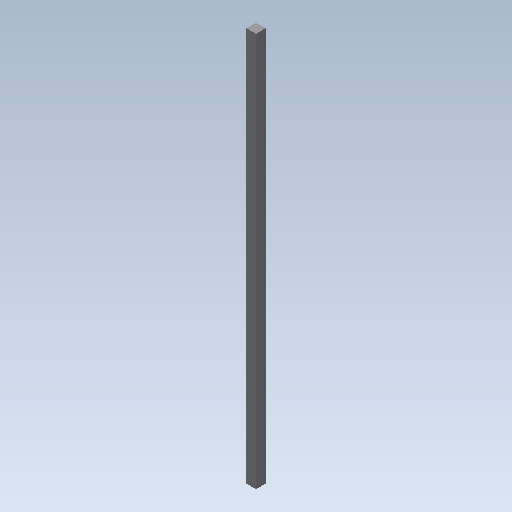
# Autodesk Inventor part: Standard
Saved by Autodesk Inventor 2020.3 (Build 243373000, 373)
## iProperties
RuleStatus: InUse
AfterDocSave0: file://Part Number Cleaner
Created: 2022-01-20
Material: Generic
Catalog Web Link: https://www.janelia.org/
Vendor: HHMI: JRC - jET
Document SubType Name: Modeling
Designer: solomone
Density: 1 g/cm^3
Appearance: Default
LAB/DEPT: A. LEE (LAB)
DESIGN DEPARTMENT: HHMI: JRC - jET
ALTERED ITEM PART NUMBER: N/A
ALTERED ITEM VENDOR: N/A
ALTERED ITEM DESCRIPTION: N/A
Title: Standard
Author: solomone
Revision Number: 0
Autodesk Inventor part; units mm, degrees
ref_plane "YZ Plane" through (0, 0, 0) normal (1, 0, 0) x (0, 1, 0)
ref_plane "XZ Plane" through (0, 0, 0) normal (0, 1, 0) x (-1, 0, 0)
ref_plane "XY Plane" through (0, 0, 0) normal (0, 0, 1) x (1, 0, 0)
sketch "Sketch1" plane through (0, 0, 0) normal (0, 1, 0) x (-1, 0, 0)
  line L0 (20, 20) -> (-20, 20)
  line L1 (-20, 20) -> (-20, -20)
  line L2 (-20, -20) -> (20, -20)
  line L3 (20, -20) -> (20, 20)
  point P0 (0, 0)
  dimension "d0" = 40
  dimension "d1" = 20
  dimension "d2" = 20
  constraints: 8 end point, 2 parallel, 2 perpendicular, 1 horizontal
  measures "d0" distance of L2.end L0.start
  measures "d1" distance from line of point (0, 0) L3
  measures "d2" distance from line of point (0, 0) L0
extrude "Extrusion1" add sketch "Sketch1" along normal blind 1651
equation "\"d1\" = 0.5 * d0"
equation "\"d2\" = d1"
body "Solid1"
